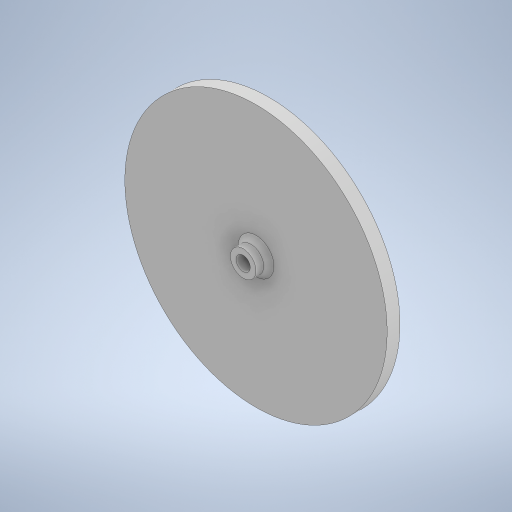
# Autodesk Inventor part: bottom
Saved by Autodesk Inventor 2023 (Build 270158000, 158)
## iProperties
Created: 2023-04-27
Part Number: bottom
Material: Generic
Document SubType Name: Modeling
Designer: alexa
Density: 1 g/cm^3
Appearance: Default
Author: alexa
Autodesk Inventor part; units mm, degrees
ref_plane "YZ Plane" through (0, 0, 0) normal (1, 0, 0) x (0, 1, 0)
ref_plane "XZ Plane" through (0, 0, 0) normal (0, 1, 0) x (-1, 0, 0)
ref_plane "XY Plane" through (0, 0, 0) normal (0, 0, 1) x (1, 0, 0)
sketch "Sketch4" plane through (0, 0, 0) normal (0, 0, 1) x (1, 0, 0)
  circle A0 centre (0, 0) radius 51.25
  circle A1 centre (0, 0) radius 2.75
  dimension "d10" = 102.5
  dimension "d11" = 5.5
  constraints: 2 centre point, 2 coincident
  measures "d10" diameter of A0
  measures "d11" diameter of A1
extrude "Extrusion4" add sketch "Sketch4" along normal blind 5
sketch "Sketch5" plane through (0, 0, 5) normal (0, 0, 1) x (1, 0, 0)
  circle A0 centre (0, 0) radius 2.75 projected
  circle A1 centre (0, 0) radius 2.75
  circle A2 centre (0, 0) radius 5
  dimension "d14" = 10
  constraints: 2 centre point, 2 coincident
  measures "d14" diameter of A2
extrude "Extrusion5" add sketch "Sketch5" along normal blind 5
chamfer "Chamfer1" distance 2 angle 45 1 edges at (-5, 0, 5)
sketch "Sketch6" plane through (0, 0, 0) normal (0, 0, -1) x (-1, 0, 0)
  circle A0 centre (0, 0) radius 2.75 projected
  circle A1 centre (0, 0) radius 2.75
  constraints: 1 centre point, 1 coincident
extrude "Extrusion6" add sketch "Sketch6" against normal blind 5
sketch "Sketch7" plane through (0, 0, 0) normal (0, 0, -1) x (-1, 0, 0)
  point P0 (0, 0)
body "Solid2"
